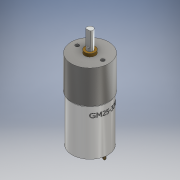
# Autodesk Inventor part: gm25-370
Saved by Autodesk Inventor 2018 (Build 220112000, 112)
## iProperties
Created: 2018-05-07
Part Number: gm25-370
Material: Generic
Document SubType Name: Modeling
Designer: aespen-cad
Density: 1 g/cm^3
Appearance: Default
Author: aespen-cad
Autodesk Inventor part; units mm, degrees
note: some values were not read from the file. Chosen so that the rebuilt part matches the saved one: direction of "Emboss1".
ref_plane "YZ Plane" through (0, 0, 0) normal (1, 0, 0) x (0, 1, 0)
ref_plane "XZ Plane" through (0, 0, 0) normal (0, 1, 0) x (-1, 0, 0)
sketch "Sketch1" plane through (0, 0, 0) normal (0, 0, 1) x (1, 0, 0)
  circle A0 centre (0, 0) radius 12
  dimension "d0" = 24
  constraints: 1 centre point, 1 coincident
  measures "d0" diameter of A0
extrude "Extrusion1" add sketch "Sketch1" along normal blind 31
fillet "Fillet1" radius 0.8 1 edges at (-12, 0, 31)
sketch "Sketch2" plane through (0, 0, 31) normal (0, 0, 1) x (1, 0, 0)
  circle A0 centre (0, 0) radius 12.5
  dimension "d4" = 25
  constraints: 1 centre point, 1 coincident
  measures "d4" diameter of A0
extrude "Extrusion2" add sketch "Sketch2" along normal blind 22
sketch "Sketch3" plane through (0, 0, 53) normal (0, 0, 1) x (1, 0, 0)
  circle A0 centre (0, 0) radius 3.5
  circle A1 centre (0, 0) radius 2.05
  dimension "d7" = 7
  dimension "d8" = 4.1
  constraints: 2 centre point, 2 coincident
  measures "d7" diameter of A0
  measures "d8" diameter of A1
extrude "Extrusion3" add sketch "Sketch3" along normal blind 2
sketch "Sketch4" plane through (0, 0, 53) normal (0, 0, 1) x (1, 0, 0)
  circle A0 centre (0, 0) radius 2.05 projected
  circle A1 centre (0, 0) radius 2
  dimension "d11" = 4
  constraints: 1 centre point, 1 coincident
  measures "d11" diameter of A1
extrude "Extrusion4" add sketch "Sketch4" along normal blind 14 contours A1
sketch "Sketch5" plane through (0, 0, 67) normal (0, 0, 1) x (1, 0, 0)
  circle A0 centre (0, 0) radius 2 projected
  line L0 (-1.4283, -1.4) -> (1.4283, -1.4)
  dimension "d14" = 3.4
  constraints: 2 end point, 2 point on circle, 1 horizontal
extrude "Extrusion5" cut sketch "Sketch5" against normal blind 10 contours L0 A0 picked at (-0.3587, -1.4953)
sketch "Sketch6" plane through (0, 0, 53) normal (0, 0, 1) x (1, 0, 0)
  circle A0 centre (-8.5, 0) radius 1.5
  circle A1 centre (8.5, 0) radius 1.5
  circle A2 centre (0, 0) radius 2.05 projected
  line L0 (-13.9622, 0) -> (14.2857, 0) construction
  dimension "d17" = 3
  dimension "d18" = 3
  dimension "d19" = 17
  dimension "d20" = 8.5
  constraints: 3 point on line, 2 centre point, 2 end point, 1 horizontal
  measures "d17" diameter of A0
  measures "d18" diameter of A1
  measures "d19" distance of A1.centre A0.centre
  measures "d20" distance of A2.centre A1.centre
hole "Hole1" at (8.5, 0, 53) at (-8.5, 0, 53) direction (0, 0, -1) diameter 2.459 depth 8.8 tip angle 118 thread size "M3x0.5" class "6H" standard "ISO Metric profile"
sketch "Sketch7" plane through (0, 0, 0) normal (0, 0, -1) x (-1, 0, 0)
  circle A0 centre (0, 0) radius 11.7
  line L0 (-9.5, 3) -> (-9.5, 3)
  line L1 (-8, 1.5) -> (-8, -1.5)
  line L2 (-9.5, -3) -> (-9.5, -3)
  line L3 (-11, -1.5) -> (-11, 1.5)
  arc A1 (-9.5, 3) -> (-11, 1.5) centre (-9.5, 1.5) ccw
  arc A2 (-8, 1.5) -> (-9.5, 3) centre (-9.5, 1.5) ccw
  arc A3 (-9.5, -3) -> (-8, -1.5) centre (-9.5, -1.5) ccw
  arc A4 (-11, -1.5) -> (-9.5, -3) centre (-9.5, -1.5) ccw
  line L4 (9.5, -3) -> (9.5, -3)
  line L5 (8, -1.5) -> (8, 1.5)
  line L6 (9.5, 3) -> (9.5, 3)
  line L7 (11, 1.5) -> (11, -1.5)
  arc A5 (9.5, -3) -> (11, -1.5) centre (9.5, -1.5) ccw
  arc A6 (8, -1.5) -> (9.5, -3) centre (9.5, -1.5) ccw
  arc A7 (9.5, 3) -> (8, 1.5) centre (9.5, 1.5) ccw
  arc A8 (11, 1.5) -> (9.5, 3) centre (9.5, 1.5) ccw
  point P0 (-8, -3)
  point P1 (-8, 3)
  point P2 (-11, -3)
  point P3 (8, 3)
  point P4 (8, -3)
  point P5 (11, 3)
  dimension "d28" = 23.4
  dimension "d29" = 3
  dimension "d30" = 6
  dimension "d31" = 3
  dimension "d32" = 8
  dimension "d33" = 1.5
  dimension "d36" = 360
  constraints: 16 end point, 16 point on circle, 12 point on line, 9 centre point, 8 tangent, 2 equal radius, 2 parallel, 1 coincident, 1 concentric, 1 horizontal, 1 perpendicular, 47 other
  measures "d28" diameter of A0
  measures "d29" distance of point (-8, -3) point (-11, -3)
  measures "d30" distance of point (-8, 3) point (-8, -3)
  measures "d31" distance from line of L0 point (0, 0)
  measures "d32" distance from line of point (0, 0) L1
  measures "d33" radius of A1
extrude "Extrusion6" cut sketch "Sketch7" against normal blind 0.4
sketch "Sketch8" plane through (0, 0, 0.4) normal (0, 0, -1) x (-1, 0, 0)
  circle A0 centre (0, 0) radius 3.25
  dimension "d40" = 6.5
  constraints: 1 centre point, 1 coincident
  measures "d40" diameter of A0
extrude "Extrusion7" add sketch "Sketch8" along normal blind 2.5
sketch "Sketch9" plane through (0, 0, 0) normal (0, 0, -1) x (-1, 0, 0)
  line L0 (-10.5, 0.2) -> (-8.5, 0.2)
  line L1 (-8.5, 0.2) -> (-8.5, -0.2)
  line L2 (-8.5, -0.2) -> (-10.5, -0.2)
  line L3 (-10.5, -0.2) -> (-10.5, 0.2)
  line L4 (8.5, 0.2) -> (10.5, 0.2)
  line L5 (10.5, 0.2) -> (10.5, -0.2)
  line L6 (10.5, -0.2) -> (8.5, -0.2)
  line L7 (8.5, -0.2) -> (8.5, 0.2)
  line L8 (-8, -1.5) -> (-8, 1.5) projected
  line L9 (8, 1.5) -> (8, -1.5) projected
  point P0 (0, 0)
  dimension "d43" = 2
  dimension "d44" = 0.4
  dimension "d45" = 2
  dimension "d46" = 0.4
  dimension "d47" = 0.5
  dimension "d48" = 0.2
  dimension "d49" = 0.2
  dimension "d50" = 0.5
  constraints: 16 end point, 4 parallel, 2 horizontal, 2 perpendicular
  measures "d43" distance of L1.end L2.end
  measures "d44" distance of L0.end L1.end
  measures "d45" distance of L5.end L6.end
  measures "d46" distance of L4.end L5.end
  measures "d47" distance between parallel lines of L8 L1
  measures "d48" distance from line of point (0, 0) L0
  measures "d49" distance from line of point (0, 0) L4
  measures "d50" distance between parallel lines of L9 L7
extrude "Extrusion8" add sketch "Sketch9" along normal blind 4
fillet "Fillet2" radius 1 6 edges at (10.5, 0, -4) (8.5, 0, -4) (-10.5, 0, -4) (-8.5, 0, -4) (3.25, 0, -2.1) (3.25, 0, 0.4)
hole "Hole2" at (9.5, -0.2, -3) direction (0, 1, 0) diameter 1 depth 8.8 tip angle 118
hole "Hole3" at (-9.5, -0.2, -3) direction (0, 1, 0) diameter 1 depth 8.8 tip angle 118
ref_plane "Work Plane1" through (12, 0, 0) normal (1, 0, 0) x (0, 1, 0)
sketch "Sketch10" plane through (12, 0, 0) normal (1, 0, 0) x (0, 1, 0)
  line L0 (-8.8686, 26.6058) -> (10.1184, 26.6058) construction
  line L1 (10.1184, 26.6058) -> (10.1184, 23.764) construction
  line L2 (10.1184, 23.764) -> (-8.8686, 23.764) construction
  line L3 (-8.8686, 23.764) -> (-8.8686, 26.6058) construction
  spline S0 degree 2 poles (-7.4119, 23.6923) (-7.7091, 23.6923) (-8.2015, 23.8739) (-8.3785, 24.0576) knots 0 0 0 1 2 2 2
  spline S1 degree 2 poles (-8.3785, 24.0576) (-8.5555, 24.2437) (-8.7438, 24.7928) (-8.7438, 25.1491) knots 0 0 0 1 2 2 2
  spline S2 degree 2 poles (-8.7438, 25.1491) (-8.7438, 25.4871) (-8.5532, 26.0226) (-8.3762, 26.2132) knots 0 0 0 1 2 2 2
  spline S3 degree 2 poles (-8.3762, 26.2132) (-8.206, 26.397) (-7.7068, 26.5967) (-7.4096, 26.5967) knots 0 0 0 1 2 2 2
  spline S4 degree 2 poles (-7.4096, 26.5967) (-7.2666, 26.5967) (-7.008, 26.5559) (-6.89, 26.5196) knots 0 0 0 1 2 2 2
  spline S5 degree 2 poles (-6.89, 26.5196) (-6.7947, 26.4923) (-6.5632, 26.3925) (-6.4929, 26.3562) knots 0 0 0 1 2 2 2
  line L4 (-6.4929, 26.3562) -> (-6.4929, 25.9069)
  line L5 (-6.4929, 25.9069) -> (-6.5247, 25.9069)
  spline S6 degree 2 poles (-6.5247, 25.9069) (-6.595, 25.9682) (-6.7425, 26.0794) (-6.8786, 26.1429) knots 0 0 0 1 2 2 2
  spline S7 degree 2 poles (-6.8786, 26.1429) (-6.9921, 26.1996) (-7.2848, 26.2745) (-7.4527, 26.2745) knots 0 0 0 1 2 2 2
  spline S8 degree 2 poles (-7.4527, 26.2745) (-7.8566, 26.2745) (-8.3558, 25.6664) (-8.3558, 25.1604) knots 0 0 0 1 2 2 2
  spline S9 degree 2 poles (-8.3558, 25.1604) (-8.3558, 24.879) (-8.2242, 24.457) (-8.0994, 24.3118) knots 0 0 0 1 2 2 2
  spline S10 degree 2 poles (-8.0994, 24.3118) (-7.9791, 24.1666) (-7.6388, 24.0145) (-7.4255, 24.0145) knots 0 0 0 1 2 2 2
  spline S11 degree 2 poles (-7.4255, 24.0145) (-7.2689, 24.0145) (-6.9558, 24.0599) (-6.8491, 24.1053) knots 0 0 0 1 2 2 2
  line L6 (-6.8491, 24.1053) -> (-6.8491, 24.8291)
  line L7 (-6.8491, 24.8291) -> (-7.4981, 24.8291)
  line L8 (-7.4981, 24.8291) -> (-7.4981, 25.1559)
  line L9 (-7.4981, 25.1559) -> (-6.4816, 25.1559)
  line L10 (-6.4816, 25.1559) -> (-6.4816, 23.9328)
  spline S12 degree 2 poles (-6.4816, 23.9328) (-6.5519, 23.9011) (-6.7924, 23.8035) (-6.8945, 23.774) knots 0 0 0 1 2 2 2
  spline S13 degree 2 poles (-6.8945, 23.774) (-7.0329, 23.7332) (-7.2553, 23.6923) (-7.4119, 23.6923) knots 0 0 0 1 2 2 2
  line L11 (-3.6135, 23.7468) -> (-3.9856, 23.7468)
  line L12 (-3.9856, 23.7468) -> (-3.9856, 26.1588)
  line L13 (-3.9856, 26.1588) -> (-4.7162, 24.5183)
  line L14 (-4.7162, 24.5183) -> (-4.9431, 24.5183)
  line L15 (-4.9431, 24.5183) -> (-5.667, 26.1588)
  line L16 (-5.667, 26.1588) -> (-5.667, 23.7468)
  line L17 (-5.667, 23.7468) -> (-6.0141, 23.7468)
  line L18 (-6.0141, 23.7468) -> (-6.0141, 26.5468)
  line L19 (-6.0141, 26.5468) -> (-5.5059, 26.5468)
  line L20 (-5.5059, 26.5468) -> (-4.807, 24.988)
  line L21 (-4.807, 24.988) -> (-4.1308, 26.5468)
  line L22 (-4.1308, 26.5468) -> (-3.6135, 26.5468)
  line L23 (-3.6135, 26.5468) -> (-3.6135, 23.7468)
  line L24 (-1.3989, 23.7468) -> (-3.1256, 23.7468)
  line L25 (-3.1256, 23.7468) -> (-3.1256, 24.1439)
  spline S14 degree 2 poles (-3.1256, 24.1439) (-2.9396, 24.3186) (-2.6083, 24.6431) (-2.4495, 24.8178) knots 0 0 0 1 2 2 2
  spline S15 degree 2 poles (-2.4495, 24.8178) (-2.1295, 25.1695) (-1.8958, 25.5915) (-1.8958, 25.8162) knots 0 0 0 1 2 2 2
  spline S16 degree 2 poles (-1.8958, 25.8162) (-1.8958, 25.9341) (-1.9684, 26.1111) (-2.0342, 26.1679) knots 0 0 0 1 2 2 2
  spline S17 degree 2 poles (-2.0342, 26.1679) (-2.1, 26.2246) (-2.2725, 26.2813) (-2.3769, 26.2813) knots 0 0 0 1 2 2 2
  spline S18 degree 2 poles (-2.3769, 26.2813) (-2.4767, 26.2813) (-2.6809, 26.2314) (-2.7739, 26.1928) knots 0 0 0 1 2 2 2
  spline S19 degree 2 poles (-2.7739, 26.1928) (-2.8534, 26.161) (-3.0008, 26.0703) (-3.0462, 26.0385) knots 0 0 0 1 2 2 2
  line L26 (-3.0462, 26.0385) -> (-3.0666, 26.0385)
  line L27 (-3.0666, 26.0385) -> (-3.0666, 26.4379)
  spline S20 degree 2 poles (-3.0666, 26.4379) (-2.9509, 26.4946) (-2.5357, 26.6058) (-2.3496, 26.6058) knots 0 0 0 1 2 2 2
  spline S21 degree 2 poles (-2.3496, 26.6058) (-1.9571, 26.6058) (-1.5146, 26.1905) (-1.5146, 25.8366) knots 0 0 0 1 2 2 2
  spline S22 degree 2 poles (-1.5146, 25.8366) (-1.5146, 25.6709) (-1.5918, 25.3941) (-1.6598, 25.2761) knots 0 0 0 1 2 2 2
  spline S23 degree 2 poles (-1.6598, 25.2761) (-1.7279, 25.1536) (-1.9253, 24.9131) (-2.0342, 24.7974) knots 0 0 0 1 2 2 2
  spline S24 degree 2 poles (-2.0342, 24.7974) (-2.2112, 24.6045) (-2.6446, 24.1915) (-2.7739, 24.0713) knots 0 0 0 1 2 2 2
  line L28 (-2.7739, 24.0713) -> (-1.3989, 24.0713)
  line L29 (-1.3989, 24.0713) -> (-1.3989, 23.7468)
  spline S25 degree 2 poles (0.6727, 24.6363) (0.6727, 24.4343) (0.5434, 24.0894) (0.4254, 23.9623) knots 0 0 0 1 2 2 2
  spline S26 degree 2 poles (0.4254, 23.9623) (0.3074, 23.8353) (-0.0443, 23.6878) (-0.2621, 23.6878) knots 0 0 0 1 2 2 2
  spline S27 degree 2 poles (-0.2621, 23.6878) (-0.4618, 23.6878) (-0.8521, 23.7763) (-0.995, 23.8466) knots 0 0 0 1 2 2 2
  line L30 (-0.995, 23.8466) -> (-0.995, 24.2437)
  line L31 (-0.995, 24.2437) -> (-0.9678, 24.2437)
  spline S28 degree 2 poles (-0.9678, 24.2437) (-0.9247, 24.2119) (-0.7636, 24.1303) (-0.666, 24.0939) knots 0 0 0 1 2 2 2
  spline S29 degree 2 poles (-0.666, 24.0939) (-0.5548, 24.0554) (-0.371, 24.0123) (-0.2553, 24.0123) knots 0 0 0 1 2 2 2
  spline S30 degree 2 poles (-0.2553, 24.0123) (-0.1418, 24.0123) (0.0714, 24.0939) (0.1486, 24.1824) knots 0 0 0 1 2 2 2
  spline S31 degree 2 poles (0.1486, 24.1824) (0.2189, 24.2664) (0.2915, 24.4888) (0.2915, 24.6385) knots 0 0 0 1 2 2 2
  spline S32 degree 2 poles (0.2915, 24.6385) (0.2915, 24.7883) (0.2099, 24.9789) (0.1327, 25.0424) knots 0 0 0 1 2 2 2
  spline S33 degree 2 poles (0.1327, 25.0424) (0.0533, 25.1127) (-0.1827, 25.1717) (-0.3256, 25.1717) knots 0 0 0 1 2 2 2
  spline S34 degree 2 poles (-0.3256, 25.1717) (-0.4799, 25.1717) (-0.7863, 25.1241) (-0.8793, 25.1037) knots 0 0 0 1 2 2 2
  line L32 (-0.8793, 25.1037) -> (-0.8793, 26.5468)
  line L33 (-0.8793, 26.5468) -> (0.6569, 26.5468)
  line L34 (0.6569, 26.5468) -> (0.6569, 26.2178)
  line L35 (0.6569, 26.2178) -> (-0.5185, 26.2178)
  line L36 (-0.5185, 26.2178) -> (-0.5185, 25.4713)
  spline S35 degree 2 poles (-0.5185, 25.4713) (-0.4504, 25.4803) (-0.3188, 25.4871) (-0.2644, 25.4871) knots 0 0 0 1 2 2 2
  spline S36 degree 2 poles (-0.2644, 25.4871) (-0.0488, 25.4871) (0.2484, 25.4168) (0.3846, 25.3124) knots 0 0 0 1 2 2 2
  spline S37 degree 2 poles (0.3846, 25.3124) (0.523, 25.208) (0.6727, 24.8904) (0.6727, 24.6363) knots 0 0 0 1 2 2 2
  line L37 (2.1022, 24.8019) -> (1.0426, 24.8019)
  line L38 (1.0426, 24.8019) -> (1.0426, 25.1422)
  line L39 (1.0426, 25.1422) -> (2.1022, 25.1422)
  line L40 (2.1022, 25.1422) -> (2.1022, 24.8019)
  spline S38 degree 2 poles (3.2299, 26.2813) (3.1278, 26.2813) (2.9259, 26.2314) (2.8283, 26.1928) knots 0 0 0 1 2 2 2
  spline S39 degree 2 poles (2.8283, 26.1928) (2.7376, 26.1542) (2.6037, 26.0726) (2.5515, 26.0363) knots 0 0 0 1 2 2 2
  line L41 (2.5515, 26.0363) -> (2.5288, 26.0363)
  line L42 (2.5288, 26.0363) -> (2.5288, 26.4333)
  spline S40 degree 2 poles (2.5288, 26.4333) (2.6513, 26.4991) (3.0711, 26.6058) (3.2594, 26.6058) knots 0 0 0 1 2 2 2
  spline S41 degree 2 poles (3.2594, 26.6058) (3.45, 26.6058) (3.7337, 26.5286) (3.8494, 26.4469) knots 0 0 0 1 2 2 2
  spline S42 degree 2 poles (3.8494, 26.4469) (3.9719, 26.3585) (4.099, 26.1021) (4.099, 25.9296) knots 0 0 0 1 2 2 2
  spline S43 degree 2 poles (4.099, 25.9296) (4.099, 25.6982) (3.7949, 25.3487) (3.5817, 25.3033) knots 0 0 0 1 2 2 2
  line L43 (3.5817, 25.3033) -> (3.5817, 25.2761)
  spline S44 degree 2 poles (3.5817, 25.2761) (3.6701, 25.258) (3.8721, 25.1763) (3.9583, 25.0946) knots 0 0 0 1 2 2 2
  spline S45 degree 2 poles (3.9583, 25.0946) (4.0445, 25.0152) (4.1534, 24.761) (4.1534, 24.5773) knots 0 0 0 1 2 2 2
  spline S46 degree 2 poles (4.1534, 24.5773) (4.1534, 24.3889) (4.0241, 24.069) (3.9061, 23.9465) knots 0 0 0 1 2 2 2
  spline S47 degree 2 poles (3.9061, 23.9465) (3.7836, 23.8194) (3.4364, 23.6878) (3.2163, 23.6878) knots 0 0 0 1 2 2 2
  spline S48 degree 2 poles (3.2163, 23.6878) (3.0053, 23.6878) (2.5923, 23.7899) (2.4517, 23.8602) knots 0 0 0 1 2 2 2
  line L44 (2.4517, 23.8602) -> (2.4517, 24.2573)
  line L45 (2.4517, 24.2573) -> (2.4789, 24.2573)
  spline S49 degree 2 poles (2.4789, 24.2573) (2.5969, 24.1711) (2.9962, 24.0123) (3.1936, 24.0123) knots 0 0 0 1 2 2 2
  spline S50 degree 2 poles (3.1936, 24.0123) (3.3094, 24.0123) (3.5408, 24.0849) (3.618, 24.1688) knots 0 0 0 1 2 2 2
  spline S51 degree 2 poles (3.618, 24.1688) (3.6928, 24.2528) (3.7723, 24.4525) (3.7723, 24.6045) knots 0 0 0 1 2 2 2
  spline S52 degree 2 poles (3.7723, 24.6045) (3.7723, 24.7565) (3.6838, 24.9539) (3.6043, 25.0106) knots 0 0 0 1 2 2 2
  spline S53 degree 2 poles (3.6043, 25.0106) (3.5249, 25.0674) (3.3094, 25.1105) (3.1823, 25.1105) knots 0 0 0 1 2 2 2
  line L46 (3.1823, 25.1105) -> (3.0235, 25.1105)
  line L47 (3.0235, 25.1105) -> (3.0235, 25.4213)
  line L48 (3.0235, 25.4213) -> (3.1483, 25.4213)
  spline S54 degree 2 poles (3.1483, 25.4213) (3.4001, 25.4213) (3.7178, 25.6619) (3.7178, 25.891) knots 0 0 0 1 2 2 2
  spline S55 degree 2 poles (3.7178, 25.891) (3.7178, 25.9977) (3.6361, 26.1497) (3.5703, 26.1951) knots 0 0 0 1 2 2 2
  spline S56 degree 2 poles (3.5703, 26.1951) (3.5, 26.2427) (3.3275, 26.2813) (3.2299, 26.2813) knots 0 0 0 1 2 2 2
  line L49 (6.334, 26.127) -> (5.1223, 23.7468)
  line L50 (5.1223, 23.7468) -> (4.723, 23.7468)
  line L51 (4.723, 23.7468) -> (6.0027, 26.2178)
  line L52 (6.0027, 26.2178) -> (4.5573, 26.2178)
  line L53 (4.5573, 26.2178) -> (4.5573, 26.5468)
  line L54 (4.5573, 26.5468) -> (6.334, 26.5468)
  line L55 (6.334, 26.5468) -> (6.334, 26.127)
  spline S57 degree 2 poles (8.4193, 25.1468) (8.4193, 24.3935) (7.9813, 23.6878) (7.5252, 23.6878) knots 0 0 0 1 2 2 2
  spline S58 degree 2 poles (7.5252, 23.6878) (7.0624, 23.6878) (6.629, 24.4071) (6.629, 25.1445) knots 0 0 0 1 2 2 2
  spline S59 degree 2 poles (6.629, 25.1445) (6.629, 25.9024) (7.0669, 26.6035) (7.5252, 26.6035) knots 0 0 0 1 2 2 2
  spline S60 degree 2 poles (7.5252, 26.6035) (7.9859, 26.6035) (8.4193, 25.8774) (8.4193, 25.1468) knots 0 0 0 1 2 2 2
  spline S61 degree 2 poles (7.9382, 24.2936) (7.9927, 24.432) (8.0381, 24.8586) (8.0381, 25.1468) knots 0 0 0 1 2 2 2
  spline S62 degree 2 poles (8.0381, 25.1468) (8.0381, 25.435) (7.9927, 25.8593) (7.9359, 26.0022) knots 0 0 0 1 2 2 2
  spline S63 degree 2 poles (7.9359, 26.0022) (7.8792, 26.1452) (7.6818, 26.2927) (7.5252, 26.2927) knots 0 0 0 1 2 2 2
  spline S64 degree 2 poles (7.5252, 26.2927) (7.3687, 26.2927) (7.1667, 26.1452) (7.1077, 25.9977) knots 0 0 0 1 2 2 2
  spline S65 degree 2 poles (7.1077, 25.9977) (7.051, 25.8547) (7.0102, 25.4191) (7.0102, 25.1445) knots 0 0 0 1 2 2 2
  spline S66 degree 2 poles (7.0102, 25.1445) (7.0102, 24.8495) (7.0465, 24.4547) (7.1055, 24.3004) knots 0 0 0 1 2 2 2
  spline S67 degree 2 poles (7.1055, 24.3004) (7.1599, 24.1552) (7.3619, 23.9986) (7.5252, 23.9986) knots 0 0 0 1 2 2 2
  spline S68 degree 2 poles (7.5252, 23.9986) (7.6795, 23.9986) (7.8815, 24.1461) (7.9382, 24.2936) knots 0 0 0 1 2 2 2
  point P0 (0, 0)
  constraints: 2 other
emboss "Emboss1" sketch "Sketch10" operation cut depth 0.2 direction (-1, 0, 0)
equation "\"d20\" = 0.5 * d19"
equation "\"d48\" = 0.5 * d44"
equation "\"d49\" = d48"
equation "\"d50\" = d47"
body "Solid1"
